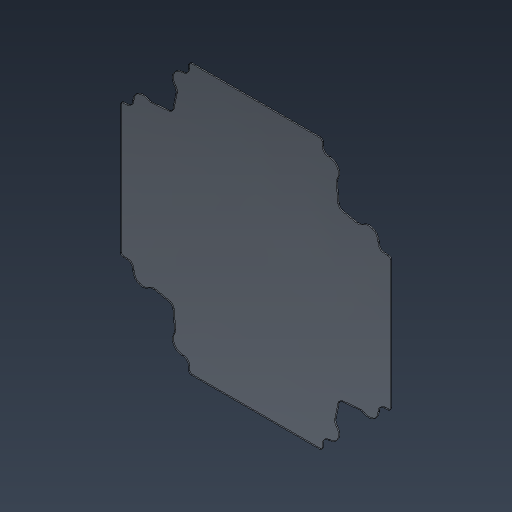
# Autodesk Inventor part: PLATE,BELLYPAN
Saved by Autodesk Inventor 2026 (Build 300175050, 175E)
## iProperties
Created: 2026-01-19
Part Number: PLATE,BELLYPAN
Material: Polycarbonate, Clear
Document SubType Name: Sheet Metal
Designer: Jthib
Mass: 1471.09 g
Surface Area: 8124.63 cm^2
Volume: 1225.91 cm^3
Density: 1.2 g/cm^3
Sheet Metal Rule: Default
Appearance: Polycarbonate - Clear
Author: Jthib
Autodesk Inventor part; units mm, degrees
ref_plane "YZ Plane" through (0, 0, 0) normal (1, 0, 0) x (0, 1, 0)
ref_plane "XZ Plane" through (0, 0, 0) normal (0, 1, 0) x (-1, 0, 0)
ref_plane "XY Plane" through (0, 0, 0) normal (0, 0, 1) x (1, 0, 0)
sketch "Sketch1" plane through (0, 0, 0) normal (0, 0, 1) x (1, 0, 0)
  line L0 (-298.45, -349.25) -> (298.45, -349.25)
  line L1 (349.25, -298.45) -> (349.25, 298.45)
  line L2 (298.45, 349.25) -> (-298.45, 349.25)
  line L3 (-349.25, 298.45) -> (-349.25, -298.45)
  line L4 (-349.25, -349.25) -> (349.25, 349.25) construction
  line L5 (349.25, -349.25) -> (-349.25, 349.25) construction
  arc A0 (349.25, 298.45) -> (298.45, 349.25) centre (298.45, 298.45) ccw
  arc A1 (-298.45, 349.25) -> (-349.25, 298.45) centre (-298.45, 298.45) ccw
  arc A2 (-349.25, -298.45) -> (-298.45, -349.25) centre (-298.45, -298.45) ccw
  arc A3 (298.45, -349.25) -> (349.25, -298.45) centre (298.45, -298.45) ccw
  point P0 (0, 0)
  dimension "d0" = 698.5
  dimension "d4" = 50.8
  measures "d0" distance of L4.end L5.end
  measures "d4" radius of A0
extrude "Plate1" add sketch "Sketch1" along normal blind 3.048
sketch "Sketch2" plane through (0, 0, 0) normal (0, 0, -1) x (-1, 0, 0)
  line L0 (-188.9125, -349.25) -> (-336.55, -349.25)
  line L1 (-179.3875, -333.375) -> (-179.3875, -339.725) construction
  arc A0 (-179.3875, -333.375) -> (-188.9125, -323.85) centre (-188.9125, -333.375) ccw construction
  line L2 (-190.5, -323.85) -> (-188.9125, -323.85) construction
  arc A1 (-221.4273, -289.3223) -> (-190.5, -323.85) centre (-190.5, -292.735) ccw construction
  arc A2 (-349.25, -336.55) -> (-336.55, -349.25) centre (-336.55, -336.55) ccw
  line L3 (-349.25, -336.55) -> (-349.25, -188.9125)
  line L4 (-339.725, -179.3875) -> (-333.375, -179.3875) construction
  arc A3 (-323.85, -188.9125) -> (-333.375, -179.3875) centre (-333.375, -188.9125) ccw construction
  line L5 (-323.85, -188.9125) -> (-323.85, -190.5) construction
  arc A4 (-323.85, -190.5) -> (-289.3223, -221.4273) centre (-292.735, -190.5) ccw construction
  arc A5 (-213.9609, -272.2965) -> (-221.4273, -289.3223) centre (-190.5, -292.735) ccw construction
  arc A6 (-213.9609, -272.2965) -> (-211.7954, -264.058) centre (-221.2002, -265.9898) ccw construction
  line L6 (-220.0695, -223.7764) -> (-211.7954, -264.058) construction
  arc A7 (-220.0695, -223.7764) -> (-224.3016, -219.9918) centre (-224.7346, -224.7346) ccw construction
  line L7 (-270.7455, -215.751) -> (-224.3016, -219.9918) construction
  arc A8 (-270.7455, -215.751) -> (-276.598, -217.1034) centre (-271.6186, -225.3124) ccw construction
  arc A9 (-289.3223, -221.4273) -> (-276.598, -217.1034) centre (-292.735, -190.5) ccw construction
  line L8 (-179.3875, -339.725) -> (-179.3875, -349.25) construction
  line L9 (-173.0375, -349.25) -> (-188.9125, -349.25)
  line L10 (-349.25, -188.9125) -> (-349.25, -173.0375)
  line L11 (-349.25, -179.3875) -> (-339.725, -179.3875) construction
  line L12 (-333.375, -173.0375) -> (-339.9898, -173.0375)
  line L13 (-339.9898, -173.0375) -> (-349.25, -173.0375)
  line L14 (-173.0375, -349.25) -> (-173.0375, -339.725)
  line L15 (-173.0375, -339.725) -> (-173.0375, -333.375)
  arc A10 (-173.0375, -333.375) -> (-188.9125, -317.5) centre (-188.9125, -333.375) ccw
  line L16 (-188.9125, -317.5) -> (-190.5, -317.5)
  arc A11 (-215.1156, -290.0188) -> (-190.5, -317.5) centre (-190.5, -292.735) ccw
  arc A12 (-209.1729, -276.4676) -> (-215.1156, -290.0188) centre (-190.5, -292.735) ccw
  arc A13 (-209.1729, -276.4676) -> (-205.5752, -262.7803) centre (-221.2002, -265.9898) ccw
  line L17 (-205.5752, -262.7803) -> (-213.8494, -222.4987)
  arc A14 (-213.8494, -222.4987) -> (-223.7241, -213.6682) centre (-224.7346, -224.7346) ccw
  line L18 (-223.7241, -213.6682) -> (-270.1681, -209.4273)
  arc A15 (-270.1681, -209.4273) -> (-279.8913, -211.6741) centre (-271.6186, -225.3124) ccw
  arc A16 (-290.0188, -215.1156) -> (-279.8913, -211.6741) centre (-292.735, -190.5) ccw
  arc A17 (-317.5, -190.5) -> (-290.0188, -215.1156) centre (-292.735, -190.5) ccw
  line L19 (-317.5, -190.5) -> (-317.5, -188.9125)
  arc A18 (-317.5, -188.9125) -> (-333.375, -173.0375) centre (-333.375, -188.9125) ccw
  line L20 (298.45, -349.25) -> (-298.45, -349.25) construction
  point P0 (0, 0)
  dimension "d9" = 6.35
  constraints: 40 end point, 38 point on circle, 19 centre point, 5 vertical, 3 horizontal, 3 perpendicular, 2 collinear, 2 point on line, 1 tangent, 55 other
  measures "d9" distance between parallel lines of L17 L6
extrude "Cut1" cut sketch "Sketch2" against normal blind 3.048
pattern_circular "Circular Pattern1" count 4 over 360 about axis through (0, 0, -10) along (0, 0, 1) of "Cut1"
fillet "Corner Round1" radius 6.35 8 edges at (349.25, -173.0375, 1.524) (173.0375, -349.25, 1.524) (-173.0375, -349.25, 1.524) (-349.25, -173.0375, 1.524) (-349.25, 173.0375, 1.524) (-173.0375, 349.25, 1.524) (173.0375, 349.25, 1.524) (349.25, 173.0375, 1.524)
equation "\"d2\" = Thickness"
equation "\"d1\" = Thickness"
equation "\"BendRadius\" = Thickness"
equation "\"BendReliefWidth\" = Thickness"
equation "\"BendReliefDepth\" = 0.5 * Thickness"
equation "\"CornerReliefSize\" = 4 * Thickness"
equation "\"MinimumRemnant\" = 2 * Thickness"
equation "\"TransitionRadius\" = BendRadius"
equation "\"JacobiRadiusSize\" = BendRadius"
equation "\"GapSize\" = Thickness"
equation "\"Thickness\" = 3.048"
body "Solid1"
